AgriRover_Cover (Autodesk Fusion 360 design; units mm, degrees)
part number: 2026-09-19-14-36-17-999
Autodesk Fusion 360 part; units mm, degrees
sketch "Sketch1" plane through (0, 0, 0) normal (0, 0, 1) x (1, 0, 0)
  line L0 (-100, 50) -> (160, 50)
  line L1 (160, 50) -> (160, -160)
  line L2 (160, -160) -> (-100, -160)
  line L3 (-100, -160) -> (-100, 50)
  dimension "d1" = 260
  dimension "d2" = 210
  constraint horizontal L0
  constraint vertical L1
  constraint horizontal L2
  constraint vertical L3
  measures "d1" distance of L0.start L0.end
  measures "d2" distance of L0.start L2.end
extrude "Extrude1" add sketch "Sketch1" along normal blind 5
fillet "Fillet1" radius 4 4 edges at (160, 50, 2.5) (160, -160, 2.5) (-100, 50, 2.5) (-100, -160, 2.5)
sketch "Sketch2" plane through (0, 0, 5) normal (0, 0, 1) x (-1, 0, 0)
  arc A0 (100, 156) -> (96, 160) centre (96, 156) ccw
  line L0 (96, 160) -> (-156, 160)
  arc A1 (-156, 160) -> (-160, 156) centre (-156, 156) ccw
  line L1 (-160, 156) -> (-160, -46)
  arc A2 (-160, -46) -> (-156, -50) centre (-156, -46) ccw
  line L2 (-156, -50) -> (96, -50)
  arc A3 (96, -50) -> (100, -46) centre (96, -46) ccw
  line L3 (100, -46) -> (100, 156)
  circle A4 centre (97, -47) radius 2
  circle A5 centre (97, 156) radius 2
  circle A6 centre (-156.5, -47) radius 2
  circle A7 centre (-156.5, 156) radius 2
  dimension "d7" = 4
  dimension "d8" = 4
  dimension "d9" = 4
  dimension "d10" = 4
  measures "d7" diameter of A4
  measures "d8" diameter of A5
  measures "d9" diameter of A6
  measures "d10" diameter of A7
extrude "Extrude2" cut sketch "Sketch2" against normal blind 5 contours A4 | A5 | A6 | A7
thread "Thread1" "ISO Metric profile 4.0 M4x0.7 M4x0.7 6H" major diameter 4.1095 minor diameter 3.332 pitch 0.7 angle 60 resizes the face on face at (-95.4679, 48.2856, 1.6667) on face at (154.5618, -156.4935, 1.6667) on face at (155.1766, 45.5004, 1.6667) on face at (-98.9382, -156.4935, 1.6667)
